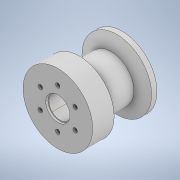
# Autodesk Inventor part: pulleyForRoundAdapter
Saved by Autodesk Inventor 2020.2 (Build 242310000, 310)
## iProperties
Created: 2020-02-15
Part Number: pulleyForRoundAdapter
Material: Generic
Document SubType Name: Modeling
Designer: robst
Density: 1 g/cm^3
Appearance: Default
Author: robst
Autodesk Inventor part; units mm, degrees
ref_plane "YZ Plane" through (0, 0, 0) normal (1, 0, 0) x (0, 1, 0)
ref_plane "XZ Plane" through (0, 0, 0) normal (0, 1, 0) x (-1, 0, 0)
ref_plane "XY Plane" through (0, 0, 0) normal (0, 0, 1) x (1, 0, 0)
sketch "Sketch1" plane through (0, 0, 0) normal (0, 0, 1) x (1, 0, 0)
  circle A0 centre (0, 0) radius 26.9875
  dimension "d0" = 53.975
  constraints: 2 coincident, 1 centre point
  measures "d0" diameter of A0
extrude "Extrusion1" add sketch "Sketch1" along normal mid plane 76.2
sketch "Sketch3" plane through (0, 0, 0) normal (1, 0, 0) x (0, 1, 0)
  line L0 (26.9875, 38.1) -> (-26.9875, 38.1) projected
  line L1 (26.9875, 38.1) -> (41.275, 38.1)
  line L2 (26.9875, -38.1) -> (26.9875, 38.1) projected
  line L3 (0, -53.34) -> (0, 53.34) projected
  line L4 (41.275, 38.1) -> (41.275, 12.7)
  line L5 (41.275, 12.7) -> (27.4636, 6.2597)
  line L6 (27.4636, 6.2597) -> (26.9875, 6.0376)
  line L7 (26.9875, -38.1) -> (26.9875, 38.1) projected
  point P0 (0, 0)
  point P1 (26.9875, 19.4779)
  point P2 (26.9875, 6.7779)
  point P3 (26.9875, 6.0376)
  dimension "d9" = 14.2875
  dimension "d12" = 25.4
  dimension "d13" = 115
  constraints: 8 end point, 2 point on line, 1 collinear, 1 horizontal, 1 vertical
  measures "d9" distance of L0.start L1.end
  measures "d12" distance of L1.end L4.end
  measures "d13" angle of L4 L5
revolve "Revolution1" add sketch "Sketch3" angle 360 about axis through (0, 0, -10) along (0, 0, 1)
sketch "Sketch4" plane through (0, 0, 0) normal (1, 0, 0) x (0, 1, 0)
  line L0 (26.9875, -38.1) -> (26.9875, 6.0376) projected
  line L1 (-26.9875, -38.1) -> (26.9875, -38.1) projected
  line L2 (26.9875, -38.1) -> (41.275, -38.1)
  line L3 (41.275, -38.1) -> (41.275, -31.75)
  line L4 (41.275, -31.75) -> (28.0457, -25.5811)
  line L5 (0, -46.7795) -> (0, 13.9768) projected
  line L6 (28.0457, -25.5811) -> (26.9875, -25.0876)
  line L7 (26.9875, -38.1) -> (26.9875, 6.0376) projected
  point P0 (0, 0)
  point P1 (26.9875, -25.8279)
  dimension "d14" = 14.2875
  dimension "d15" = 6.35
  dimension "d16" = 115
  constraints: 8 end point, 1 collinear, 1 horizontal, 1 perpendicular, 1 point on line
  measures "d14" distance of L0.start L2.end
  measures "d15" distance of L2.end L3.end
  measures "d16" angle of L4 L3
revolve "Revolution2" add sketch "Sketch4" angle 360 about axis through (0, 0, -10) along (0, 0, 1)
sketch "Sketch5" plane through (0, 0, 38.1) normal (0, 0, 1) x (1, 0, 0)
  circle A0 centre (0, 0) radius 13.0969
  dimension "d18" = 26.1938
  constraints: 1 centre point, 1 coincident
  measures "d18" diameter of A0
extrude "Extrusion4" cut sketch "Sketch5" against normal blind 25.4
sketch "Sketch6" plane through (0, 0, 38.1) normal (0, 0, 1) x (1, 0, 0)
  circle A0 centre (0, 0) radius 14.2875
  dimension "d21" = 28.575
  constraints: 1 centre point, 1 coincident
  measures "d21" diameter of A0
extrude "Extrusion5" cut sketch "Sketch6" against normal blind 2.54
mirror "Mirror2" about plane through (0, 0, 0) normal (0, 0, 1) of "Extrusion5", "Extrusion4"
sketch "Sketch7" plane through (0, 0, 38.1) normal (0, 0, 1) x (1, 0, 0)
  circle A0 centre (0, 23.8125) radius 2.5527
  circle A1 centre (-20.6222, 11.9063) radius 2.5527
  circle A2 centre (-20.6222, -11.9062) radius 2.5527
  circle A3 centre (0, -23.8125) radius 2.5527
  circle A4 centre (20.6222, -11.9063) radius 2.5527
  circle A5 centre (20.6222, 11.9062) radius 2.5527
  point P0 (0, 0)
  dimension "d24" = 5.1054
  dimension "d27" = 360
  dimension "d29" = 23.8125
  constraints: 6 centre point, 13 other
  measures "d24" diameter of A0
  measures "d29" distance of A0.centre point (0, 0)
extrude "Extrusion6" cut sketch "Sketch7" against normal through all
body "Solid1"
